Autodesk Fusion 360 part; units mm, degrees
note: some values were not read from the file. Chosen so that the rebuilt part matches the saved one: a direction. Set by a fixed rule: which sketch regions a step uses.
(part 7 of 8)
sketch "Sketch8" plane through (0, 65.3924, 0) normal (0, 1, 0) x (-1, 0, 0)
  arc A0 (-58.6914, 4.8735) -> (-58.96, 3.871) centre (-53.7044, 3) ccw
  arc A1 (-59.0732, 3.7884) -> (-58.96, 3.871) centre (-59.0587, 3.8873) ccw
  line L0 (-59.0732, 3.7884) -> (-59.8406, 3.9011)
  spline S0 degree 5 poles (-59.8406, 3.9011) (-59.8449, 3.9017) (-59.8536, 3.9029) (-59.8668, 3.9042) (-59.8844, 3.9051) (-59.9064, 3.9052) (-59.9286, 3.9045) (-59.9508, 3.9033) (-59.973, 3.9019) (-59.9953, 3.9002) (-60.0176, 3.8984) (-60.0399, 3.8963) (-60.0622, 3.8939) (-60.0846, 3.8912) (-60.107, 3.888) (-60.1294, 3.8845) (-60.1518, 3.8806) (-60.1743, 3.8765) (-60.1967, 3.8722) (-60.2192, 3.8676) (-60.2417, 3.8629) (-60.2641, 3.8579) (-60.2866, 3.8526) (-60.3091, 3.8471) (-60.3316, 3.8414) (-60.3541, 3.8354) (-60.3766, 3.8292) (-60.3991, 3.8228) (-60.4216, 3.8162) (-60.4441, 3.8093) (-60.4666, 3.8023) (-60.4891, 3.795) (-60.5116, 3.7876) (-60.5341, 3.7799) (-60.5565, 3.7721) (-60.579, 3.764) (-60.6014, 3.7558) (-60.6239, 3.7474) (-60.6463, 3.7387) (-60.6687, 3.7299) (-60.6912, 3.7209) (-60.7135, 3.7117) (-60.7359, 3.7023) (-60.7583, 3.6928) (-60.7806, 3.683) (-60.803, 3.6731) (-60.8253, 3.663) (-60.8476, 3.6527) (-60.8699, 3.6423) (-60.8921, 3.6317) (-60.9144, 3.6209) (-60.9366, 3.6099) (-60.9588, 3.5988) (-60.9809, 3.5874) (-61.0031, 3.576) (-61.0252, 3.5643) (-61.0473, 3.5525) (-61.0694, 3.5405) (-61.0914, 3.5284) (-61.1134, 3.516) (-61.1354, 3.5036) (-61.1574, 3.4909) (-61.1793, 3.4781) (-61.2012, 3.4652) (-61.2231, 3.452) (-61.2449, 3.4388) (-61.2667, 3.4253) (-61.2885, 3.4117) (-61.3102, 3.398) (-61.3319, 3.3841) (-61.3536, 3.37) (-61.3709, 3.3586) (-61.3839, 3.35) (-61.3925, 3.3443) (-61.3968, 3.3414) knots 0 0 0 0 0 0 0.01428571 0.02857143 0.04285714 0.05714286 0.07142857 0.08571429 0.1 0.11428571 0.12857143 0.14285714 0.15714286 0.17142857 0.18571429 0.2 0.21428571 0.22857143 0.24285714 0.25714286 0.27142857 0.28571429 0.3 0.31428571 0.32857143 0.34285714 0.35714286 0.37142857 0.38571429 0.4 0.41428571 0.42857143 0.44285714 0.45714286 0.47142857 0.48571429 0.5 0.51428571 0.52857143 0.54285714 0.55714286 0.57142857 0.58571429 0.6 0.61428571 0.62857143 0.64285714 0.65714286 0.67142857 0.68571429 0.7 0.71428571 0.72857143 0.74285714 0.75714286 0.77142857 0.78571429 0.8 0.81428571 0.82857143 0.84285714 0.85714286 0.87142857 0.88571429 0.9 0.91428571 0.92857143 0.94285714 0.95714286 0.97142857 0.98571429 1 1 1 1 1 1
  arc A2 (-61.3968, 3.3414) -> (-61.3968, 2.6586) centre (-53.7044, 3) ccw
  spline S1 degree 5 poles (-61.3968, 2.6586) (-61.3925, 2.6557) (-61.3839, 2.65) (-61.3709, 2.6414) (-61.3536, 2.63) (-61.3319, 2.6159) (-61.3102, 2.602) (-61.2885, 2.5883) (-61.2667, 2.5747) (-61.2449, 2.5612) (-61.2231, 2.548) (-61.2012, 2.5348) (-61.1793, 2.5219) (-61.1574, 2.5091) (-61.1354, 2.4964) (-61.1134, 2.484) (-61.0914, 2.4716) (-61.0694, 2.4595) (-61.0473, 2.4475) (-61.0252, 2.4357) (-61.0031, 2.424) (-60.9809, 2.4126) (-60.9588, 2.4012) (-60.9366, 2.3901) (-60.9144, 2.3791) (-60.8921, 2.3683) (-60.8699, 2.3577) (-60.8476, 2.3473) (-60.8253, 2.337) (-60.803, 2.3269) (-60.7806, 2.317) (-60.7583, 2.3072) (-60.7359, 2.2977) (-60.7135, 2.2883) (-60.6912, 2.2791) (-60.6687, 2.2701) (-60.6463, 2.2613) (-60.6239, 2.2526) (-60.6014, 2.2442) (-60.579, 2.236) (-60.5565, 2.2279) (-60.5341, 2.2201) (-60.5116, 2.2124) (-60.4891, 2.205) (-60.4666, 2.1977) (-60.4441, 2.1907) (-60.4216, 2.1838) (-60.3991, 2.1772) (-60.3766, 2.1708) (-60.3541, 2.1646) (-60.3316, 2.1586) (-60.3091, 2.1529) (-60.2866, 2.1474) (-60.2641, 2.1421) (-60.2417, 2.1371) (-60.2192, 2.1324) (-60.1967, 2.1278) (-60.1743, 2.1235) (-60.1518, 2.1194) (-60.1294, 2.1155) (-60.107, 2.112) (-60.0846, 2.1088) (-60.0622, 2.1061) (-60.0399, 2.1037) (-60.0176, 2.1016) (-59.9953, 2.0998) (-59.973, 2.0981) (-59.9508, 2.0967) (-59.9286, 2.0955) (-59.9064, 2.0948) (-59.8844, 2.0949) (-59.8668, 2.0958) (-59.8536, 2.0971) (-59.8449, 2.0983) (-59.8406, 2.0989) knots -1 -1 -1 -1 -1 -1 -0.98571429 -0.97142857 -0.95714286 -0.94285714 -0.92857143 -0.91428571 -0.9 -0.88571429 -0.87142857 -0.85714286 -0.84285714 -0.82857143 -0.81428571 -0.8 -0.78571429 -0.77142857 -0.75714286 -0.74285714 -0.72857143 -0.71428571 -0.7 -0.68571429 -0.67142857 -0.65714286 -0.64285714 -0.62857143 -0.61428571 -0.6 -0.58571429 -0.57142857 -0.55714286 -0.54285714 -0.52857143 -0.51428571 -0.5 -0.48571429 -0.47142857 -0.45714286 -0.44285714 -0.42857143 -0.41428571 -0.4 -0.38571429 -0.37142857 -0.35714286 -0.34285714 -0.32857143 -0.31428571 -0.3 -0.28571429 -0.27142857 -0.25714286 -0.24285714 -0.22857143 -0.21428571 -0.2 -0.18571429 -0.17142857 -0.15714286 -0.14285714 -0.12857143 -0.11428571 -0.1 -0.08571429 -0.07142857 -0.05714286 -0.04285714 -0.02857143 -0.01428571 0 0 0 0 0 0
  line L1 (-59.8406, 2.0989) -> (-59.0732, 2.2116)
  arc A3 (-58.96, 2.129) -> (-59.0732, 2.2116) centre (-59.0587, 2.1127) ccw
  arc A4 (-58.96, 2.129) -> (-58.6914, 1.1265) centre (-53.7044, 3) ccw
  arc A5 (-58.7481, 0.9984) -> (-58.6914, 1.1265) centre (-58.785, 1.0913) ccw
  line L2 (-58.7481, 0.9984) -> (-59.469, 0.7123)
  spline S2 degree 5 poles (-59.469, 0.7123) (-59.4731, 0.7106) (-59.4812, 0.7073) (-59.4933, 0.7018) (-59.5089, 0.6938) (-59.5281, 0.6829) (-59.5469, 0.6712) (-59.5656, 0.6591) (-59.5841, 0.6467) (-59.6026, 0.6342) (-59.621, 0.6215) (-59.6393, 0.6085) (-59.6574, 0.5953) (-59.6754, 0.5817) (-59.6932, 0.5677) (-59.7108, 0.5535) (-59.7283, 0.5389) (-59.7457, 0.5241) (-59.763, 0.5092) (-59.7802, 0.494) (-59.7973, 0.4786) (-59.8142, 0.463) (-59.8311, 0.4473) (-59.8478, 0.4313) (-59.8644, 0.415) (-59.8809, 0.3986) (-59.8973, 0.382) (-59.9136, 0.3652) (-59.9298, 0.3482) (-59.9458, 0.331) (-59.9618, 0.3137) (-59.9776, 0.2962) (-59.9934, 0.2785) (-60.009, 0.2606) (-60.0246, 0.2426) (-60.04, 0.2244) (-60.0553, 0.206) (-60.0705, 0.1875) (-60.0856, 0.1688) (-60.1006, 0.1499) (-60.1156, 0.1309) (-60.1304, 0.1118) (-60.145, 0.0925) (-60.1596, 0.073) (-60.1741, 0.0534) (-60.1885, 0.0336) (-60.2028, 0.0137) (-60.217, -0.0063) (-60.231, -0.0265) (-60.245, -0.0468) (-60.2588, -0.0673) (-60.2726, -0.0879) (-60.2862, -0.1087) (-60.2998, -0.1295) (-60.3132, -0.1506) (-60.3266, -0.1717) (-60.3398, -0.193) (-60.3529, -0.2144) (-60.3659, -0.2359) (-60.3788, -0.2576) (-60.3916, -0.2794) (-60.4043, -0.3013) (-60.4169, -0.3234) (-60.4294, -0.3456) (-60.4418, -0.3679) (-60.4541, -0.3903) (-60.4662, -0.4128) (-60.4783, -0.4355) (-60.4902, -0.4583) (-60.5021, -0.4812) (-60.5138, -0.5042) (-60.5231, -0.5227) (-60.53, -0.5366) (-60.5346, -0.5459) (-60.5369, -0.5506) knots 0 0 0 0 0 0 0.01428571 0.02857143 0.04285714 0.05714286 0.07142857 0.08571429 0.1 0.11428571 0.12857143 0.14285714 0.15714286 0.17142857 0.18571429 0.2 0.21428571 0.22857143 0.24285714 0.25714286 0.27142857 0.28571429 0.3 0.31428571 0.32857143 0.34285714 0.35714286 0.37142857 0.38571429 0.4 0.41428571 0.42857143 0.44285714 0.45714286 0.47142857 0.48571429 0.5 0.51428571 0.52857143 0.54285714 0.55714286 0.57142857 0.58571429 0.6 0.61428571 0.62857143 0.64285714 0.65714286 0.67142857 0.68571429 0.7 0.71428571 0.72857143 0.74285714 0.75714286 0.77142857 0.78571429 0.8 0.81428571 0.82857143 0.84285714 0.85714286 0.87142857 0.88571429 0.9 0.91428571 0.92857143 0.94285714 0.95714286 0.97142857 0.98571429 1 1 1 1 1 1
  arc A6 (-60.5369, -0.5506) -> (-60.1955, -1.1419) centre (-53.7044, 3) ccw
  spline S3 degree 5 poles (-60.1955, -1.1419) (-60.1904, -1.1422) (-60.18, -1.1429) (-60.1645, -1.1438) (-60.1438, -1.145) (-60.118, -1.1464) (-60.0922, -1.1476) (-60.0665, -1.1486) (-60.0409, -1.1495) (-60.0153, -1.1502) (-59.9897, -1.1508) (-59.9642, -1.1513) (-59.9388, -1.1515) (-59.9134, -1.1516) (-59.8881, -1.1516) (-59.8628, -1.1514) (-59.8376, -1.1511) (-59.8124, -1.1506) (-59.7873, -1.1499) (-59.7622, -1.1491) (-59.7373, -1.1481) (-59.7123, -1.147) (-59.6875, -1.1457) (-59.6627, -1.1443) (-59.638, -1.1427) (-59.6133, -1.1409) (-59.5887, -1.139) (-59.5642, -1.1369) (-59.5398, -1.1346) (-59.5154, -1.1322) (-59.4911, -1.1297) (-59.4669, -1.1269) (-59.4427, -1.124) (-59.4186, -1.1209) (-59.3947, -1.1177) (-59.3707, -1.1143) (-59.3469, -1.1107) (-59.3232, -1.107) (-59.2995, -1.1031) (-59.2759, -1.099) (-59.2525, -1.0947) (-59.2291, -1.0903) (-59.2058, -1.0857) (-59.1826, -1.0809) (-59.1595, -1.0759) (-59.1365, -1.0708) (-59.1136, -1.0654) (-59.0908, -1.0599) (-59.0681, -1.0542) (-59.0455, -1.0483) (-59.023, -1.0423) (-59.0007, -1.036) (-58.9785, -1.0295) (-58.9564, -1.0228) (-58.9344, -1.0159) (-58.9126, -1.0088) (-58.8908, -1.0015) (-58.8692, -0.994) (-58.8477, -0.9864) (-58.8264, -0.9785) (-58.8052, -0.9703) (-58.7842, -0.9619) (-58.7635, -0.9531) (-58.7429, -0.944) (-58.7226, -0.9346) (-58.7023, -0.9251) (-58.6823, -0.9154) (-58.6623, -0.9055) (-58.6425, -0.8954) (-58.6229, -0.8849) (-58.6039, -0.8738) (-58.5891, -0.8642) (-58.5784, -0.8565) (-58.5714, -0.8512) (-58.5679, -0.8484) knots -1 -1 -1 -1 -1 -1 -0.98571429 -0.97142857 -0.95714286 -0.94285714 -0.92857143 -0.91428571 -0.9 -0.88571429 -0.87142857 -0.85714286 -0.84285714 -0.82857143 -0.81428571 -0.8 -0.78571429 -0.77142857 -0.75714286 -0.74285714 -0.72857143 -0.71428571 -0.7 -0.68571429 -0.67142857 -0.65714286 -0.64285714 -0.62857143 -0.61428571 -0.6 -0.58571429 -0.57142857 -0.55714286 -0.54285714 -0.52857143 -0.51428571 -0.5 -0.48571429 -0.47142857 -0.45714286 -0.44285714 -0.42857143 -0.41428571 -0.4 -0.38571429 -0.37142857 -0.35714286 -0.34285714 -0.32857143 -0.31428571 -0.3 -0.28571429 -0.27142857 -0.25714286 -0.24285714 -0.22857143 -0.21428571 -0.2 -0.18571429 -0.17142857 -0.15714286 -0.14285714 -0.12857143 -0.11428571 -0.1 -0.08571429 -0.07142857 -0.05714286 -0.04285714 -0.02857143 -0.01428571 0 0 0 0 0 0
  line L3 (-58.5679, -0.8484) -> (-57.9597, -0.3672)
  arc A7 (-57.8204, -0.3821) -> (-57.9597, -0.3672) centre (-57.8977, -0.4456) ccw
  arc A8 (-57.8204, -0.3821) -> (-57.0865, -1.116) centre (-53.7044, 3) ccw
  arc A9 (-57.0716, -1.2553) -> (-57.0865, -1.116) centre (-57.15, -1.1933) ccw
  line L4 (-57.0716, -1.2553) -> (-57.5528, -1.8635)
  spline S4 degree 5 poles (-57.5528, -1.8635) (-57.5556, -1.867) (-57.5609, -1.874) (-57.5686, -1.8847) (-57.5782, -1.8995) (-57.5893, -1.9185) (-57.5998, -1.9381) (-57.6099, -1.9579) (-57.6197, -1.9779) (-57.6295, -1.998) (-57.639, -2.0182) (-57.6484, -2.0385) (-57.6575, -2.0591) (-57.6663, -2.0798) (-57.6747, -2.1008) (-57.6829, -2.122) (-57.6908, -2.1433) (-57.6984, -2.1648) (-57.7059, -2.1864) (-57.7132, -2.2082) (-57.7203, -2.23) (-57.7272, -2.252) (-57.7339, -2.2741) (-57.7404, -2.2963) (-57.7467, -2.3187) (-57.7527, -2.3411) (-57.7586, -2.3637) (-57.7643, -2.3864) (-57.7698, -2.4092) (-57.7751, -2.4321) (-57.7803, -2.4551) (-57.7853, -2.4782) (-57.7901, -2.5014) (-57.7947, -2.5247) (-57.7991, -2.5481) (-57.8034, -2.5716) (-57.8075, -2.5951) (-57.8114, -2.6188) (-57.8151, -2.6425) (-57.8187, -2.6664) (-57.8221, -2.6903) (-57.8253, -2.7143) (-57.8284, -2.7383) (-57.8313, -2.7625) (-57.834, -2.7867) (-57.8366, -2.811) (-57.839, -2.8354) (-57.8413, -2.8598) (-57.8434, -2.8843) (-57.8453, -2.9089) (-57.8471, -2.9336) (-57.8487, -2.9583) (-57.8501, -2.9831) (-57.8514, -3.008) (-57.8525, -3.0329) (-57.8535, -3.0579) (-57.8543, -3.0829) (-57.855, -3.108) (-57.8555, -3.1332) (-57.8558, -3.1584) (-57.856, -3.1837) (-57.856, -3.209) (-57.8559, -3.2344) (-57.8556, -3.2599) (-57.8552, -3.2854) (-57.8546, -3.3109) (-57.8539, -3.3365) (-57.853, -3.3622) (-57.852, -3.3879) (-57.8508, -3.4136) (-57.8494, -3.4394) (-57.8482, -3.4601) (-57.8473, -3.4756) (-57.8466, -3.486) (-57.8462, -3.4911) knots 0 0 0 0 0 0 0.01428571 0.02857143 0.04285714 0.05714286 0.07142857 0.08571429 0.1 0.11428571 0.12857143 0.14285714 0.15714286 0.17142857 0.18571429 0.2 0.21428571 0.22857143 0.24285714 0.25714286 0.27142857 0.28571429 0.3 0.31428571 0.32857143 0.34285714 0.35714286 0.37142857 0.38571429 0.4 0.41428571 0.42857143 0.44285714 0.45714286 0.47142857 0.48571429 0.5 0.51428571 0.52857143 0.54285714 0.55714286 0.57142857 0.58571429 0.6 0.61428571 0.62857143 0.64285714 0.65714286 0.67142857 0.68571429 0.7 0.71428571 0.72857143 0.74285714 0.75714286 0.77142857 0.78571429 0.8 0.81428571 0.82857143 0.84285714 0.85714286 0.87142857 0.88571429 0.9 0.91428571 0.92857143 0.94285714 0.95714286 0.97142857 0.98571429 1 1 1 1 1 1
  arc A10 (-57.8462, -3.4911) -> (-57.255, -3.8325) centre (-53.7044, 3) ccw
  spline S5 degree 5 poles (-57.255, -3.8325) (-57.2503, -3.8302) (-57.241, -3.8256) (-57.2271, -3.8187) (-57.2086, -3.8094) (-57.1855, -3.7977) (-57.1626, -3.7858) (-57.1399, -3.7739) (-57.1172, -3.7618) (-57.0947, -3.7497) (-57.0723, -3.7374) (-57.05, -3.725) (-57.0278, -3.7125) (-57.0057, -3.6999) (-56.9838, -3.6872) (-56.962, -3.6744) (-56.9403, -3.6615) (-56.9188, -3.6485) (-56.8974, -3.6354) (-56.8761, -3.6222) (-56.8549, -3.6088) (-56.8339, -3.5954) (-56.813, -3.5819) (-56.7923, -3.5682) (-56.7717, -3.5545) (-56.7512, -3.5406) (-56.7309, -3.5266) (-56.7107, -3.5126) (-56.6906, -3.4984) (-56.6707, -3.4841) (-56.651, -3.4697) (-56.6314, -3.4552) (-56.6119, -3.4407) (-56.5926, -3.426) (-56.5735, -3.4112) (-56.5544, -3.3963) (-56.5356, -3.3813) (-56.5169, -3.3661) (-56.4984, -3.3509) (-56.48, -3.3356) (-56.4618, -3.3202) (-56.4438, -3.3046) (-56.4259, -3.289) (-56.4082, -3.2732) (-56.3907, -3.2574) (-56.3734, -3.2414) (-56.3562, -3.2254) (-56.3392, -3.2092) (-56.3224, -3.1929) (-56.3058, -3.1765) (-56.2893, -3.16) (-56.2731, -3.1434) (-56.2571, -3.1267) (-56.2413, -3.1098) (-56.2258, -3.0929) (-56.2104, -3.0758) (-56.1952, -3.0586) (-56.1802, -3.0413) (-56.1655, -3.024) (-56.1509, -3.0065) (-56.1367, -2.9888) (-56.1227, -2.971) (-56.1091, -2.953) (-56.0959, -2.9349) (-56.0829, -2.9166) (-56.0702, -2.8982) (-56.0577, -2.8797) (-56.0453, -2.8612) (-56.0332, -2.8426) (-56.0215, -2.8237) (-56.0105, -2.8046) (-56.0026, -2.7889) (-55.9971, -2.7768) (-55.9937, -2.7687) (-55.9921, -2.7646) knots -1 -1 -1 -1 -1 -1 -0.98571429 -0.97142857 -0.95714286 -0.94285714 -0.92857143 -0.91428571 -0.9 -0.88571429 -0.87142857 -0.85714286 -0.84285714 -0.82857143 -0.81428571 -0.8 -0.78571429 -0.77142857 -0.75714286 -0.74285714 -0.72857143 -0.71428571 -0.7 -0.68571429 -0.67142857 -0.65714286 -0.64285714 -0.62857143 -0.61428571 -0.6 -0.58571429 -0.57142857 -0.55714286 -0.54285714 -0.52857143 -0.51428571 -0.5 -0.48571429 -0.47142857 -0.45714286 -0.44285714 -0.42857143 -0.41428571 -0.4 -0.38571429 -0.37142857 -0.35714286 -0.34285714 -0.32857143 -0.31428571 -0.3 -0.28571429 -0.27142857 -0.25714286 -0.24285714 -0.22857143 -0.21428571 -0.2 -0.18571429 -0.17142857 -0.15714286 -0.14285714 -0.12857143 -0.11428571 -0.1 -0.08571429 -0.07142857 -0.05714286 -0.04285714 -0.02857143 -0.01428571 0 0 0 0 0 0
  line L5 (-55.9921, -2.7646) -> (-55.706, -2.0437)
  arc A11 (-55.5779, -1.987) -> (-55.706, -2.0437) centre (-55.6131, -2.0806) ccw
  arc A12 (-55.5779, -1.987) -> (-54.5754, -2.2556) centre (-53.7044, 3) ccw
  arc A13 (-54.4928, -2.3688) -> (-54.5754, -2.2556) centre (-54.5917, -2.3543) ccw
  line L6 (-54.4928, -2.3688) -> (-54.6055, -3.1362)
  spline S6 degree 5 poles (-54.6055, -3.1362) (-54.6061, -3.1405) (-54.6072, -3.1493) (-54.6085, -3.1624) (-54.6095, -3.18) (-54.6096, -3.202) (-54.6089, -3.2242) (-54.6077, -3.2464) (-54.6063, -3.2686) (-54.6046, -3.2909) (-54.6028, -3.3132) (-54.6007, -3.3355) (-54.5983, -3.3578) (-54.5956, -3.3802) (-54.5924, -3.4026) (-54.5889, -3.425) (-54.585, -3.4474) (-54.5809, -3.4699) (-54.5766, -3.4923) (-54.572, -3.5148) (-54.5672, -3.5373) (-54.5622, -3.5598) (-54.557, -3.5822) (-54.5515, -3.6047) (-54.5458, -3.6272) (-54.5398, -3.6497) (-54.5336, -3.6722) (-54.5272, -3.6947) (-54.5205, -3.7172) (-54.5137, -3.7397) (-54.5067, -3.7622) (-54.4994, -3.7847) (-54.492, -3.8072) (-54.4843, -3.8297) (-54.4765, -3.8521) (-54.4684, -3.8746) (-54.4602, -3.8971) (-54.4517, -3.9195) (-54.4431, -3.9419) (-54.4343, -3.9644) (-54.4253, -3.9868) (-54.4161, -4.0092) (-54.4067, -4.0315) (-54.3972, -4.0539) (-54.3874, -4.0763) (-54.3775, -4.0986) (-54.3674, -4.1209) (-54.3571, -4.1432) (-54.3467, -4.1655) (-54.3361, -4.1877) (-54.3253, -4.21) (-54.3143, -4.2322) (-54.3031, -4.2544) (-54.2918, -4.2765) (-54.2803, -4.2987) (-54.2687, -4.3208) (-54.2569, -4.3429) (-54.2449, -4.365) (-54.2327, -4.387) (-54.2204, -4.409) (-54.208, -4.431) (-54.1953, -4.453) (-54.1825, -4.4749) (-54.1696, -4.4968) (-54.1564, -4.5187) (-54.1432, -4.5405) (-54.1297, -4.5623) (-54.1161, -4.5841) (-54.1024, -4.6058) (-54.0885, -4.6275) (-54.0744, -4.6492) (-54.063, -4.6665) (-54.0544, -4.6795) (-54.0487, -4.6881) (-54.0458, -4.6924) knots 0 0 0 0 0 0 0.01428571 0.02857143 0.04285714 0.05714286 0.07142857 0.08571429 0.1 0.11428571 0.12857143 0.14285714 0.15714286 0.17142857 0.18571429 0.2 0.21428571 0.22857143 0.24285714 0.25714286 0.27142857 0.28571429 0.3 0.31428571 0.32857143 0.34285714 0.35714286 0.37142857 0.38571429 0.4 0.41428571 0.42857143 0.44285714 0.45714286 0.47142857 0.48571429 0.5 0.51428571 0.52857143 0.54285714 0.55714286 0.57142857 0.58571429 0.6 0.61428571 0.62857143 0.64285714 0.65714286 0.67142857 0.68571429 0.7 0.71428571 0.72857143 0.74285714 0.75714286 0.77142857 0.78571429 0.8 0.81428571 0.82857143 0.84285714 0.85714286 0.87142857 0.88571429 0.9 0.91428571 0.92857143 0.94285714 0.95714286 0.97142857 0.98571429 1 1 1 1 1 1
  arc A14 (-54.0458, -4.6924) -> (-53.363, -4.6924) centre (-53.7044, 3) ccw
  spline S7 degree 5 poles (-53.363, -4.6924) (-53.3601, -4.6881) (-53.3544, -4.6795) (-53.3458, -4.6665) (-53.3344, -4.6492) (-53.3203, -4.6275) (-53.3064, -4.6058) (-53.2927, -4.5841) (-53.2791, -4.5623) (-53.2656, -4.5405) (-53.2523, -4.5187) (-53.2392, -4.4968) (-53.2263, -4.4749) (-53.2135, -4.453) (-53.2008, -4.431) (-53.1883, -4.409) (-53.176, -4.387) (-53.1639, -4.365) (-53.1519, -4.3429) (-53.1401, -4.3208) (-53.1284, -4.2987) (-53.117, -4.2765) (-53.1056, -4.2544) (-53.0945, -4.2322) (-53.0835, -4.21) (-53.0727, -4.1877) (-53.0621, -4.1655) (-53.0516, -4.1432) (-53.0414, -4.1209) (-53.0313, -4.0986) (-53.0213, -4.0763) (-53.0116, -4.0539) (-53.0021, -4.0315) (-52.9927, -4.0092) (-52.9835, -3.9868) (-52.9745, -3.9644) (-52.9657, -3.9419) (-52.957, -3.9195) (-52.9486, -3.8971) (-52.9403, -3.8746) (-52.9323, -3.8521) (-52.9244, -3.8297) (-52.9168, -3.8072) (-52.9093, -3.7847) (-52.9021, -3.7622) (-52.8951, -3.7397) (-52.8882, -3.7172) (-52.8816, -3.6947) (-52.8752, -3.6722) (-52.869, -3.6497) (-52.863, -3.6272) (-52.8573, -3.6047) (-52.8518, -3.5822) (-52.8465, -3.5598) (-52.8415, -3.5373) (-52.8368, -3.5148) (-52.8322, -3.4923) (-52.8279, -3.4699) (-52.8238, -3.4474) (-52.8199, -3.425) (-52.8164, -3.4026) (-52.8132, -3.3802) (-52.8104, -3.3578) (-52.808, -3.3355) (-52.806, -3.3132) (-52.8042, -3.2909) (-52.8025, -3.2686) (-52.8011, -3.2464) (-52.7999, -3.2242) (-52.7992, -3.202) (-52.7993, -3.18) (-52.8002, -3.1624) (-52.8015, -3.1493) (-52.8027, -3.1405) (-52.8033, -3.1362) knots -1 -1 -1 -1 -1 -1 -0.98571429 -0.97142857 -0.95714286 -0.94285714 -0.92857143 -0.91428571 -0.9 -0.88571429 -0.87142857 -0.85714286 -0.84285714 -0.82857143 -0.81428571 -0.8 -0.78571429 -0.77142857 -0.75714286 -0.74285714 -0.72857143 -0.71428571 -0.7 -0.68571429 -0.67142857 -0.65714286 -0.64285714 -0.62857143 -0.61428571 -0.6 -0.58571429 -0.57142857 -0.55714286 -0.54285714 -0.52857143 -0.51428571 -0.5 -0.48571429 -0.47142857 -0.45714286 -0.44285714 -0.42857143 -0.41428571 -0.4 -0.38571429 -0.37142857 -0.35714286 -0.34285714 -0.32857143 -0.31428571 -0.3 -0.28571429 -0.27142857 -0.25714286 -0.24285714 -0.22857143 -0.21428571 -0.2 -0.18571429 -0.17142857 -0.15714286 -0.14285714 -0.12857143 -0.11428571 -0.1 -0.08571429 -0.07142857 -0.05714286 -0.04285714 -0.02857143 -0.01428571 0 0 0 0 0 0
  line L7 (-52.8033, -3.1362) -> (-52.916, -2.3688)
  arc A15 (-52.8334, -2.2556) -> (-52.916, -2.3688) centre (-52.8171, -2.3543) ccw
  arc A16 (-52.8334, -2.2556) -> (-51.8309, -1.987) centre (-53.7044, 3) ccw
  arc A17 (-51.7028, -2.0437) -> (-51.8309, -1.987) centre (-51.7957, -2.0806) ccw
  line L8 (-51.7028, -2.0437) -> (-51.4167, -2.7646)
  spline S8 degree 5 poles (-51.4167, -2.7646) (-51.415, -2.7687) (-51.4117, -2.7768) (-51.4062, -2.7889) (-51.3982, -2.8046) (-51.3873, -2.8237) (-51.3756, -2.8426) (-51.3635, -2.8612) (-51.3511, -2.8797) (-51.3386, -2.8982) (-51.3258, -2.9166) (-51.3129, -2.9349) (-51.2997, -2.953) (-51.2861, -2.971) (-51.2721, -2.9888) (-51.2579, -3.0065) (-51.2433, -3.024) (-51.2285, -3.0413) (-51.2135, -3.0586) (-51.1984, -3.0758) (-51.183, -3.0929) (-51.1674, -3.1098) (-51.1517, -3.1267) (-51.1356, -3.1434) (-51.1194, -3.16) (-51.103, -3.1765) (-51.0864, -3.1929) (-51.0696, -3.2092) (-51.0526, -3.2254) (-51.0354, -3.2414) (-51.0181, -3.2574) (-51.0006, -3.2732) (-50.9829, -3.289) (-50.965, -3.3046) (-50.947, -3.3202) (-50.9288, -3.3356) (-50.9104, -3.3509) (-50.8919, -3.3661) (-50.8732, -3.3813) (-50.8543, -3.3963) (-50.8353, -3.4112) (-50.8162, -3.426) (-50.7969, -3.4407) (-50.7774, -3.4552) (-50.7578, -3.4697) (-50.738, -3.4841) (-50.7181, -3.4984) (-50.6981, -3.5126) (-50.6779, -3.5266) (-50.6576, -3.5406) (-50.6371, -3.5545) (-50.6165, -3.5682) (-50.5957, -3.5819) (-50.5749, -3.5954) (-50.5538, -3.6088) (-50.5327, -3.6222) (-50.5114, -3.6354) (-50.49, -3.6485) (-50.4684, -3.6615) (-50.4468, -3.6744) (-50.425, -3.6872) (-50.403, -3.6999) (-50.381, -3.7125) (-50.3588, -3.725) (-50.3365, -3.7374) (-50.3141, -3.7497) (-50.2916, -3.7618) (-50.2689, -3.7739) (-50.2461, -3.7858) (-50.2232, -3.7977) (-50.2002, -3.8094) (-50.1817, -3.8187) (-50.1678, -3.8256) (-50.1585, -3.8302) (-50.1538, -3.8325) knots 0 0 0 0 0 0 0.01428571 0.02857143 0.04285714 0.05714286 0.07142857 0.08571429 0.1 0.11428571 0.12857143 0.14285714 0.15714286 0.17142857 0.18571429 0.2 0.21428571 0.22857143 0.24285714 0.25714286 0.27142857 0.28571429 0.3 0.31428571 0.32857143 0.34285714 0.35714286 0.37142857 0.38571429 0.4 0.41428571 0.42857143 0.44285714 0.45714286 0.47142857 0.48571429 0.5 0.51428571 0.52857143 0.54285714 0.55714286 0.57142857 0.58571429 0.6 0.61428571 0.62857143 0.64285714 0.65714286 0.67142857 0.68571429 0.7 0.71428571 0.72857143 0.74285714 0.75714286 0.77142857 0.78571429 0.8 0.81428571 0.82857143 0.84285714 0.85714286 0.87142857 0.88571429 0.9 0.91428571 0.92857143 0.94285714 0.95714286 0.97142857 0.98571429 1 1 1 1 1 1
  arc A18 (-50.1538, -3.8325) -> (-49.5625, -3.4911) centre (-53.7044, 3) ccw
  spline S9 degree 5 poles (-49.5625, -3.4911) (-49.5622, -3.486) (-49.5615, -3.4756) (-49.5605, -3.4601) (-49.5593, -3.4394) (-49.558, -3.4136) (-49.5568, -3.3879) (-49.5558, -3.3622) (-49.5549, -3.3365) (-49.5541, -3.3109) (-49.5536, -3.2854) (-49.5531, -3.2599) (-49.5529, -3.2344) (-49.5527, -3.209) (-49.5528, -3.1837) (-49.553, -3.1584) (-49.5533, -3.1332) (-49.5538, -3.108) (-49.5545, -3.0829) (-49.5553, -3.0579) (-49.5562, -3.0329) (-49.5574, -3.008) (-49.5587, -2.9831) (-49.5601, -2.9583) (-49.5617, -2.9336) (-49.5635, -2.9089) (-49.5654, -2.8843) (-49.5675, -2.8598) (-49.5697, -2.8354) (-49.5722, -2.811) (-49.5747, -2.7867) (-49.5775, -2.7625) (-49.5804, -2.7383) (-49.5834, -2.7143) (-49.5867, -2.6903) (-49.5901, -2.6664) (-49.5937, -2.6425) (-49.5974, -2.6188) (-49.6013, -2.5951) (-49.6054, -2.5716) (-49.6097, -2.5481) (-49.6141, -2.5247) (-49.6187, -2.5014) (-49.6235, -2.4782) (-49.6285, -2.4551) (-49.6336, -2.4321) (-49.639, -2.4092) (-49.6445, -2.3864) (-49.6502, -2.3637) (-49.656, -2.3411) (-49.6621, -2.3187) (-49.6684, -2.2963) (-49.6749, -2.2741) (-49.6816, -2.252) (-49.6885, -2.23) (-49.6956, -2.2082) (-49.7029, -2.1864) (-49.7104, -2.1648) (-49.718, -2.1433) (-49.7259, -2.122) (-49.7341, -2.1008) (-49.7425, -2.0798) (-49.7513, -2.0591) (-49.7604, -2.0385) (-49.7697, -2.0182) (-49.7793, -1.998) (-49.789, -1.9779) (-49.7989, -1.9579) (-49.809, -1.9381) (-49.8195, -1.9185) (-49.8306, -1.8995) (-49.8402, -1.8847) (-49.8479, -1.874) (-49.8532, -1.867) (-49.856, -1.8635) knots -1 -1 -1 -1 -1 -1 -0.98571429 -0.97142857 -0.95714286 -0.94285714 -0.92857143 -0.91428571 -0.9 -0.88571429 -0.87142857 -0.85714286 -0.84285714 -0.82857143 -0.81428571 -0.8 -0.78571429 -0.77142857 -0.75714286 -0.74285714 -0.72857143 -0.71428571 -0.7 -0.68571429 -0.67142857 -0.65714286 -0.64285714 -0.62857143 -0.61428571 -0.6 -0.58571429 -0.57142857 -0.55714286 -0.54285714 -0.52857143 -0.51428571 -0.5 -0.48571429 -0.47142857 -0.45714286 -0.44285714 -0.42857143 -0.41428571 -0.4 -0.38571429 -0.37142857 -0.35714286 -0.34285714 -0.32857143 -0.31428571 -0.3 -0.28571429 -0.27142857 -0.25714286 -0.24285714 -0.22857143 -0.21428571 -0.2 -0.18571429 -0.17142857 -0.15714286 -0.14285714 -0.12857143 -0.11428571 -0.1 -0.08571429 -0.07142857 -0.05714286 -0.04285714 -0.02857143 -0.01428571 0 0 0 0 0 0
  line L9 (-49.856, -1.8635) -> (-50.3372, -1.2553)
  arc A19 (-50.3223, -1.116) -> (-50.3372, -1.2553) centre (-50.2588, -1.1933) ccw
  arc A20 (-50.3223, -1.116) -> (-49.5884, -0.3821) centre (-53.7044, 3) ccw
  arc A21 (-49.4491, -0.3672) -> (-49.5884, -0.3821) centre (-49.5111, -0.4456) ccw
  line L10 (-49.4491, -0.3672) -> (-48.8409, -0.8484)
  spline S10 degree 5 poles (-48.8409, -0.8484) (-48.8374, -0.8512) (-48.8304, -0.8565) (-48.8197, -0.8642) (-48.8049, -0.8738) (-48.7859, -0.8849) (-48.7663, -0.8954) (-48.7465, -0.9055) (-48.7265, -0.9154) (-48.7064, -0.9251) (-48.6862, -0.9346) (-48.6659, -0.944) (-48.6453, -0.9531) (-48.6246, -0.9619) (-48.6036, -0.9703) (-48.5824, -0.9785) (-48.5611, -0.9864) (-48.5396, -0.994) (-48.5179, -1.0015) (-48.4962, -1.0088) (-48.4744, -1.0159) (-48.4524, -1.0228) (-48.4303, -1.0295) (-48.4081, -1.036) (-48.3857, -1.0423) (-48.3633, -1.0483) (-48.3407, -1.0542) (-48.318, -1.0599) (-48.2952, -1.0654) (-48.2723, -1.0708) (-48.2493, -1.0759) (-48.2262, -1.0809) (-48.203, -1.0857) (-48.1797, -1.0903) (-48.1563, -1.0947) (-48.1328, -1.099) (-48.1093, -1.1031) (-48.0856, -1.107) (-48.0619, -1.1107) (-48.038, -1.1143) (-48.0141, -1.1177) (-47.9901, -1.1209) (-47.9661, -1.124) (-47.9419, -1.1269) (-47.9177, -1.1297) (-47.8934, -1.1322) (-47.869, -1.1346) (-47.8446, -1.1369) (-47.8201, -1.139) (-47.7955, -1.1409) (-47.7708, -1.1427) (-47.7461, -1.1443) (-47.7213, -1.1457) (-47.6964, -1.147) (-47.6715, -1.1481) (-47.6465, -1.1491) (-47.6215, -1.1499) (-47.5964, -1.1506) (-47.5712, -1.1511) (-47.546, -1.1514) (-47.5207, -1.1516) (-47.4954, -1.1516) (-47.47, -1.1515) (-47.4445, -1.1513) (-47.419, -1.1508) (-47.3935, -1.1502) (-47.3679, -1.1495) (-47.3422, -1.1486) (-47.3165, -1.1476) (-47.2908, -1.1464) (-47.265, -1.145) (-47.2443, -1.1438) (-47.2288, -1.1429) (-47.2184, -1.1422) (-47.2132, -1.1419) knots 0 0 0 0 0 0 0.01428571 0.02857143 0.04285714 0.05714286 0.07142857 0.08571429 0.1 0.11428571 0.12857143 0.14285714 0.15714286 0.17142857 0.18571429 0.2 0.21428571 0.22857143 0.24285714 0.25714286 0.27142857 0.28571429 0.3 0.31428571 0.32857143 0.34285714 0.35714286 0.37142857 0.38571429 0.4 0.41428571 0.42857143 0.44285714 0.45714286 0.47142857 0.48571429 0.5 0.51428571 0.52857143 0.54285714 0.55714286 0.57142857 0.58571429 0.6 0.61428571 0.62857143 0.64285714 0.65714286 0.67142857 0.68571429 0.7 0.71428571 0.72857143 0.74285714 0.75714286 0.77142857 0.78571429 0.8 0.81428571 0.82857143 0.84285714 0.85714286 0.87142857 0.88571429 0.9 0.91428571 0.92857143 0.94285714 0.95714286 0.97142857 0.98571429 1 1 1 1 1 1
  arc A22 (-47.2132, -1.1419) -> (-46.8719, -0.5506) centre (-53.7044, 3) ccw
  spline S11 degree 5 poles (-46.8719, -0.5506) (-46.8742, -0.5459) (-46.8787, -0.5366) (-46.8857, -0.5227) (-46.895, -0.5042) (-46.9067, -0.4812) (-46.9186, -0.4583) (-46.9305, -0.4355) (-46.9426, -0.4128) (-46.9547, -0.3903) (-46.967, -0.3679) (-46.9794, -0.3456) (-46.9919, -0.3234) (-47.0044, -0.3013) (-47.0171, -0.2794) (-47.0299, -0.2576) (-47.0429, -0.2359) (-47.0559, -0.2144) (-47.069, -0.193) (-47.0822, -0.1717) (-47.0956, -0.1506) (-47.109, -0.1295) (-47.1225, -0.1087) (-47.1362, -0.0879) (-47.1499, -0.0673) (-47.1638, -0.0468) (-47.1778, -0.0265) (-47.1918, -0.0063) (-47.206, 0.0137) (-47.2203, 0.0336) (-47.2347, 0.0534) (-47.2491, 0.073) (-47.2637, 0.0925) (-47.2784, 0.1118) (-47.2932, 0.1309) (-47.3081, 0.1499) (-47.3231, 0.1688) (-47.3382, 0.1875) (-47.3535, 0.206) (-47.3688, 0.2244) (-47.3842, 0.2426) (-47.3997, 0.2606) (-47.4154, 0.2785) (-47.4311, 0.2962) (-47.447, 0.3137) (-47.463, 0.331) (-47.479, 0.3482) (-47.4952, 0.3652) (-47.5115, 0.382) (-47.5279, 0.3986) (-47.5443, 0.415) (-47.561, 0.4313) (-47.5777, 0.4473) (-47.5945, 0.463) (-47.6115, 0.4786) (-47.6286, 0.494) (-47.6458, 0.5092) (-47.663, 0.5241) (-47.6804, 0.5389) (-47.6979, 0.5535) (-47.7156, 0.5677) (-47.7334, 0.5817) (-47.7514, 0.5953) (-47.7695, 0.6085) (-47.7878, 0.6215) (-47.8062, 0.6342) (-47.8247, 0.6467) (-47.8432, 0.6591) (-47.8618, 0.6712) (-47.8807, 0.6829) (-47.8998, 0.6938) (-47.9155, 0.7018) (-47.9275, 0.7073) (-47.9357, 0.7106) (-47.9398, 0.7123) knots -1 -1 -1 -1 -1 -1 -0.98571429 -0.97142857 -0.95714286 -0.94285714 -0.92857143 -0.91428571 -0.9 -0.88571429 -0.87142857 -0.85714286 -0.84285714 -0.82857143 -0.81428571 -0.8 -0.78571429 -0.77142857 -0.75714286 -0.74285714 -0.72857143 -0.71428571 -0.7 -0.68571429 -0.67142857 -0.65714286 -0.64285714 -0.62857143 -0.61428571 -0.6 -0.58571429 -0.57142857 -0.55714286 -0.54285714 -0.52857143 -0.51428571 -0.5 -0.48571429 -0.47142857 -0.45714286 -0.44285714 -0.42857143 -0.41428571 -0.4 -0.38571429 -0.37142857 -0.35714286 -0.34285714 -0.32857143 -0.31428571 -0.3 -0.28571429 -0.27142857 -0.25714286 -0.24285714 -0.22857143 -0.21428571 -0.2 -0.18571429 -0.17142857 -0.15714286 -0.14285714 -0.12857143 -0.11428571 -0.1 -0.08571429 -0.07142857 -0.05714286 -0.04285714 -0.02857143 -0.01428571 0 0 0 0 0 0
  line L11 (-47.9398, 0.7123) -> (-48.6607, 0.9984)
  arc A23 (-48.7174, 1.1265) -> (-48.6607, 0.9984) centre (-48.6238, 1.0913) ccw
  arc A24 (-48.7174, 1.1265) -> (-48.4488, 2.129) centre (-53.7044, 3) ccw
  arc A25 (-48.3356, 2.2116) -> (-48.4488, 2.129) centre (-48.3501, 2.1127) ccw
  line L12 (-48.3356, 2.2116) -> (-47.5682, 2.0989)
  spline S12 degree 5 poles (-47.5682, 2.0989) (-47.5639, 2.0983) (-47.5551, 2.0971) (-47.542, 2.0958) (-47.5244, 2.0949) (-47.5023, 2.0948) (-47.4802, 2.0955) (-47.458, 2.0967) (-47.4358, 2.0981) (-47.4135, 2.0998) (-47.3912, 2.1016) (-47.3689, 2.1037) (-47.3465, 2.1061) (-47.3242, 2.1088) (-47.3018, 2.112) (-47.2794, 2.1155) (-47.2569, 2.1194) (-47.2345, 2.1235) (-47.212, 2.1278) (-47.1896, 2.1324) (-47.1671, 2.1371) (-47.1446, 2.1421) (-47.1221, 2.1474) (-47.0997, 2.1529) (-47.0772, 2.1586) (-47.0547, 2.1646) (-47.0322, 2.1708) (-47.0097, 2.1772) (-46.9872, 2.1838) (-46.9647, 2.1907) (-46.9422, 2.1977) (-46.9197, 2.205) (-46.8972, 2.2124) (-46.8747, 2.2201) (-46.8523, 2.2279) (-46.8298, 2.236) (-46.8073, 2.2442) (-46.7849, 2.2526) (-46.7625, 2.2613) (-46.74, 2.2701) (-46.7176, 2.2791) (-46.6952, 2.2883) (-46.6729, 2.2977) (-46.6505, 2.3072) (-46.6281, 2.317) (-46.6058, 2.3269) (-46.5835, 2.337) (-46.5612, 2.3473) (-46.5389, 2.3577) (-46.5167, 2.3683) (-46.4944, 2.3791) (-46.4722, 2.3901) (-46.45, 2.4012) (-46.4278, 2.4126) (-46.4057, 2.424) (-46.3836, 2.4357) (-46.3615, 2.4475) (-46.3394, 2.4595) (-46.3174, 2.4716) (-46.2953, 2.484) (-46.2734, 2.4964) (-46.2514, 2.5091) (-46.2295, 2.5219) (-46.2076, 2.5348) (-46.1857, 2.548) (-46.1639, 2.5612) (-46.1421, 2.5747) (-46.1203, 2.5883) (-46.0986, 2.602) (-46.0769, 2.6159) (-46.0552, 2.63) (-46.0379, 2.6414) (-46.0249, 2.65) (-46.0163, 2.6557) (-46.012, 2.6586) knots 0 0 0 0 0 0 0.01428571 0.02857143 0.04285714 0.05714286 0.07142857 0.08571429 0.1 0.11428571 0.12857143 0.14285714 0.15714286 0.17142857 0.18571429 0.2 0.21428571 0.22857143 0.24285714 0.25714286 0.27142857 0.28571429 0.3 0.31428571 0.32857143 0.34285714 0.35714286 0.37142857 0.38571429 0.4 0.41428571 0.42857143 0.44285714 0.45714286 0.47142857 0.48571429 0.5 0.51428571 0.52857143 0.54285714 0.55714286 0.57142857 0.58571429 0.6 0.61428571 0.62857143 0.64285714 0.65714286 0.67142857 0.68571429 0.7 0.71428571 0.72857143 0.74285714 0.75714286 0.77142857 0.78571429 0.8 0.81428571 0.82857143 0.84285714 0.85714286 0.87142857 0.88571429 0.9 0.91428571 0.92857143 0.94285714 0.95714286 0.97142857 0.98571429 1 1 1 1 1 1
  arc A26 (-46.012, 2.6586) -> (-46.012, 3.3414) centre (-53.7044, 3) ccw
  spline S13 degree 5 poles (-46.012, 3.3414) (-46.0163, 3.3443) (-46.0249, 3.35) (-46.0379, 3.3586) (-46.0552, 3.37) (-46.0769, 3.3841) (-46.0986, 3.398) (-46.1203, 3.4117) (-46.1421, 3.4253) (-46.1639, 3.4388) (-46.1857, 3.452) (-46.2076, 3.4652) (-46.2295, 3.4781) (-46.2514, 3.4909) (-46.2734, 3.5036) (-46.2953, 3.516) (-46.3174, 3.5284) (-46.3394, 3.5405) (-46.3615, 3.5525) (-46.3836, 3.5643) (-46.4057, 3.576) (-46.4278, 3.5874) (-46.45, 3.5988) (-46.4722, 3.6099) (-46.4944, 3.6209) (-46.5167, 3.6317) (-46.5389, 3.6423) (-46.5612, 3.6527) (-46.5835, 3.663) (-46.6058, 3.6731) (-46.6281, 3.683) (-46.6505, 3.6928) (-46.6729, 3.7023) (-46.6952, 3.7117) (-46.7176, 3.7209) (-46.74, 3.7299) (-46.7625, 3.7387) (-46.7849, 3.7474) (-46.8073, 3.7558) (-46.8298, 3.764) (-46.8523, 3.7721) (-46.8747, 3.7799) (-46.8972, 3.7876) (-46.9197, 3.795) (-46.9422, 3.8023) (-46.9647, 3.8093) (-46.9872, 3.8162) (-47.0097, 3.8228) (-47.0322, 3.8292) (-47.0547, 3.8354) (-47.0772, 3.8414) (-47.0997, 3.8471) (-47.1221, 3.8526) (-47.1446, 3.8579) (-47.1671, 3.8629) (-47.1896, 3.8676) (-47.212, 3.8722) (-47.2345, 3.8765) (-47.2569, 3.8806) (-47.2794, 3.8845) (-47.3018, 3.888) (-47.3242, 3.8912) (-47.3465, 3.8939) (-47.3689, 3.8963) (-47.3912, 3.8984) (-47.4135, 3.9002) (-47.4358, 3.9019) (-47.458, 3.9033) (-47.4802, 3.9045) (-47.5023, 3.9052) (-47.5244, 3.9051) (-47.542, 3.9042) (-47.5551, 3.9029) (-47.5639, 3.9017) (-47.5682, 3.9011) knots -1 -1 -1 -1 -1 -1 -0.98571429 -0.97142857 -0.95714286 -0.94285714 -0.92857143 -0.91428571 -0.9 -0.88571429 -0.87142857 -0.85714286 -0.84285714 -0.82857143 -0.81428571 -0.8 -0.78571429 -0.77142857 -0.75714286 -0.74285714 -0.72857143 -0.71428571 -0.7 -0.68571429 -0.67142857 -0.65714286 -0.64285714 -0.62857143 -0.61428571 -0.6 -0.58571429 -0.57142857 -0.55714286 -0.54285714 -0.52857143 -0.51428571 -0.5 -0.48571429 -0.47142857 -0.45714286 -0.44285714 -0.42857143 -0.41428571 -0.4 -0.38571429 -0.37142857 -0.35714286 -0.34285714 -0.32857143 -0.31428571 -0.3 -0.28571429 -0.27142857 -0.25714286 -0.24285714 -0.22857143 -0.21428571 -0.2 -0.18571429 -0.17142857 -0.15714286 -0.14285714 -0.12857143 -0.11428571 -0.1 -0.08571429 -0.07142857 -0.05714286 -0.04285714 -0.02857143 -0.01428571 0 0 0 0 0 0
  line L13 (-47.5682, 3.9011) -> (-48.3356, 3.7884)
  arc A27 (-48.4488, 3.871) -> (-48.3356, 3.7884) centre (-48.3501, 3.8873) ccw
  arc A28 (-48.4488, 3.871) -> (-48.7174, 4.8735) centre (-53.7044, 3) ccw
  arc A29 (-48.6607, 5.0016) -> (-48.7174, 4.8735) centre (-48.6238, 4.9087) ccw
  line L14 (-48.6607, 5.0016) -> (-47.9398, 5.2877)
  spline S14 degree 5 poles (-47.9398, 5.2877) (-47.9357, 5.2894) (-47.9275, 5.2927) (-47.9155, 5.2982) (-47.8998, 5.3062) (-47.8807, 5.3171) (-47.8618, 5.3288) (-47.8432, 5.3409) (-47.8247, 5.3533) (-47.8062, 5.3658) (-47.7878, 5.3785) (-47.7695, 5.3915) (-47.7514, 5.4047) (-47.7334, 5.4183) (-47.7156, 5.4323) (-47.6979, 5.4465) (-47.6804, 5.4611) (-47.663, 5.4759) (-47.6458, 5.4908) (-47.6286, 5.506) (-47.6115, 5.5214) (-47.5945, 5.537) (-47.5777, 5.5527) (-47.561, 5.5687) (-47.5443, 5.585) (-47.5279, 5.6014) (-47.5115, 5.618) (-47.4952, 5.6348) (-47.479, 5.6518) (-47.463, 5.669) (-47.447, 5.6863) (-47.4311, 5.7038) (-47.4154, 5.7215) (-47.3997, 5.7394) (-47.3842, 5.7574) (-47.3688, 5.7756) (-47.3535, 5.794) (-47.3382, 5.8125) (-47.3231, 5.8312) (-47.3081, 5.8501) (-47.2932, 5.8691) (-47.2784, 5.8882) (-47.2637, 5.9075) (-47.2491, 5.927) (-47.2347, 5.9466) (-47.2203, 5.9664) (-47.206, 5.9863) (-47.1918, 6.0063) (-47.1778, 6.0265) (-47.1638, 6.0468) (-47.1499, 6.0673) (-47.1362, 6.0879) (-47.1225, 6.1087) (-47.109, 6.1295) (-47.0956, 6.1506) (-47.0822, 6.1717) (-47.069, 6.193) (-47.0559, 6.2144) (-47.0429, 6.2359) (-47.0299, 6.2576) (-47.0171, 6.2794) (-47.0044, 6.3013) (-46.9919, 6.3234) (-46.9794, 6.3456) (-46.967, 6.3679) (-46.9547, 6.3903) (-46.9426, 6.4128) (-46.9305, 6.4355) (-46.9186, 6.4583) (-46.9067, 6.4812) (-46.895, 6.5042) (-46.8857, 6.5227) (-46.8787, 6.5366) (-46.8742, 6.5459) (-46.8719, 6.5506) knots 0 0 0 0 0 0 0.01428571 0.02857143 0.04285714 0.05714286 0.07142857 0.08571429 0.1 0.11428571 0.12857143 0.14285714 0.15714286 0.17142857 0.18571429 0.2 0.21428571 0.22857143 0.24285714 0.25714286 0.27142857 0.28571429 0.3 0.31428571 0.32857143 0.34285714 0.35714286 0.37142857 0.38571429 0.4 0.41428571 0.42857143 0.44285714 0.45714286 0.47142857 0.48571429 0.5 0.51428571 0.52857143 0.54285714 0.55714286 0.57142857 0.58571429 0.6 0.61428571 0.62857143 0.64285714 0.65714286 0.67142857 0.68571429 0.7 0.71428571 0.72857143 0.74285714 0.75714286 0.77142857 0.78571429 0.8 0.81428571 0.82857143 0.84285714 0.85714286 0.87142857 0.88571429 0.9 0.91428571 0.92857143 0.94285714 0.95714286 0.97142857 0.98571429 1 1 1 1 1 1
  arc A30 (-46.8719, 6.5506) -> (-47.2132, 7.1419) centre (-53.7044, 3) ccw
  spline S15 degree 5 poles (-47.2132, 7.1419) (-47.2184, 7.1422) (-47.2288, 7.1429) (-47.2443, 7.1438) (-47.265, 7.145) (-47.2908, 7.1464) (-47.3165, 7.1476) (-47.3422, 7.1486) (-47.3679, 7.1495) (-47.3935, 7.1502) (-47.419, 7.1508) (-47.4445, 7.1513) (-47.47, 7.1515) (-47.4954, 7.1516) (-47.5207, 7.1516) (-47.546, 7.1514) (-47.5712, 7.1511) (-47.5964, 7.1506) (-47.6215, 7.1499) (-47.6465, 7.1491) (-47.6715, 7.1481) (-47.6964, 7.147) (-47.7213, 7.1457) (-47.7461, 7.1443) (-47.7708, 7.1427) (-47.7955, 7.1409) (-47.8201, 7.139) (-47.8446, 7.1369) (-47.869, 7.1346) (-47.8934, 7.1322) (-47.9177, 7.1297) (-47.9419, 7.1269) (-47.9661, 7.124) (-47.9901, 7.1209) (-48.0141, 7.1177) (-48.038, 7.1143) (-48.0619, 7.1107) (-48.0856, 7.107) (-48.1093, 7.1031) (-48.1328, 7.099) (-48.1563, 7.0947) (-48.1797, 7.0903) (-48.203, 7.0857) (-48.2262, 7.0809) (-48.2493, 7.0759) (-48.2723, 7.0708) (-48.2952, 7.0654) (-48.318, 7.0599) (-48.3407, 7.0542) (-48.3633, 7.0483) (-48.3857, 7.0423) (-48.4081, 7.036) (-48.4303, 7.0295) (-48.4524, 7.0228) (-48.4744, 7.0159) (-48.4962, 7.0088) (-48.5179, 7.0015) (-48.5396, 6.994) (-48.5611, 6.9864) (-48.5824, 6.9785) (-48.6036, 6.9703) (-48.6246, 6.9619) (-48.6453, 6.9531) (-48.6659, 6.944) (-48.6862, 6.9346) (-48.7064, 6.9251) (-48.7265, 6.9154) (-48.7465, 6.9055) (-48.7663, 6.8954) (-48.7859, 6.8849) (-48.8049, 6.8738) (-48.8197, 6.8642) (-48.8304, 6.8565) (-48.8374, 6.8512) (-48.8409, 6.8484) knots -1 -1 -1 -1 -1 -1 -0.98571429 -0.97142857 -0.95714286 -0.94285714 -0.92857143 -0.91428571 -0.9 -0.88571429 -0.87142857 -0.85714286 -0.84285714 -0.82857143 -0.81428571 -0.8 -0.78571429 -0.77142857 -0.75714286 -0.74285714 -0.72857143 -0.71428571 -0.7 -0.68571429 -0.67142857 -0.65714286 -0.64285714 -0.62857143 -0.61428571 -0.6 -0.58571429 -0.57142857 -0.55714286 -0.54285714 -0.52857143 -0.51428571 -0.5 -0.48571429 -0.47142857 -0.45714286 -0.44285714 -0.42857143 -0.41428571 -0.4 -0.38571429 -0.37142857 -0.35714286 -0.34285714 -0.32857143 -0.31428571 -0.3 -0.28571429 -0.27142857 -0.25714286 -0.24285714 -0.22857143 -0.21428571 -0.2 -0.18571429 -0.17142857 -0.15714286 -0.14285714 -0.12857143 -0.11428571 -0.1 -0.08571429 -0.07142857 -0.05714286 -0.04285714 -0.02857143 -0.01428571 0 0 0 0 0 0
  line L15 (-48.8409, 6.8484) -> (-49.4491, 6.3672)
  arc A31 (-49.5884, 6.3821) -> (-49.4491, 6.3672) centre (-49.5111, 6.4456) ccw
  arc A32 (-49.5884, 6.3821) -> (-50.3223, 7.116) centre (-53.7044, 3) ccw
  arc A33 (-50.3372, 7.2553) -> (-50.3223, 7.116) centre (-50.2588, 7.1933) ccw
  line L16 (-50.3372, 7.2553) -> (-49.856, 7.8635)
  spline S16 degree 5 poles (-49.856, 7.8635) (-49.8532, 7.867) (-49.8479, 7.874) (-49.8402, 7.8847) (-49.8306, 7.8995) (-49.8195, 7.9185) (-49.809, 7.9381) (-49.7989, 7.9579) (-49.789, 7.9779) (-49.7793, 7.998) (-49.7697, 8.0182) (-49.7604, 8.0385) (-49.7513, 8.0591) (-49.7425, 8.0798) (-49.7341, 8.1008) (-49.7259, 8.122) (-49.718, 8.1433) (-49.7104, 8.1648) (-49.7029, 8.1864) (-49.6956, 8.2082) (-49.6885, 8.23) (-49.6816, 8.252) (-49.6749, 8.2741) (-49.6684, 8.2963) (-49.6621, 8.3187) (-49.656, 8.3411) (-49.6502, 8.3637) (-49.6445, 8.3864) (-49.639, 8.4092) (-49.6336, 8.4321) (-49.6285, 8.4551) (-49.6235, 8.4782) (-49.6187, 8.5014) (-49.6141, 8.5247) (-49.6097, 8.5481) (-49.6054, 8.5716) (-49.6013, 8.5951) (-49.5974, 8.6188) (-49.5937, 8.6425) (-49.5901, 8.6664) (-49.5867, 8.6903) (-49.5834, 8.7143) (-49.5804, 8.7383) (-49.5775, 8.7625) (-49.5747, 8.7867) (-49.5722, 8.811) (-49.5697, 8.8354) (-49.5675, 8.8598) (-49.5654, 8.8843) (-49.5635, 8.9089) (-49.5617, 8.9336) (-49.5601, 8.9583) (-49.5587, 8.9831) (-49.5574, 9.008) (-49.5562, 9.0329) (-49.5553, 9.0579) (-49.5545, 9.0829) (-49.5538, 9.108) (-49.5533, 9.1332) (-49.553, 9.1584) (-49.5528, 9.1837) (-49.5527, 9.209) (-49.5529, 9.2344) (-49.5531, 9.2599) (-49.5536, 9.2854) (-49.5541, 9.3109) (-49.5549, 9.3365) (-49.5558, 9.3622) (-49.5568, 9.3879) (-49.558, 9.4136) (-49.5593, 9.4394) (-49.5605, 9.4601) (-49.5615, 9.4756) (-49.5622, 9.486) (-49.5625, 9.4911) knots 0 0 0 0 0 0 0.01428571 0.02857143 0.04285714 0.05714286 0.07142857 0.08571429 0.1 0.11428571 0.12857143 0.14285714 0.15714286 0.17142857 0.18571429 0.2 0.21428571 0.22857143 0.24285714 0.25714286 0.27142857 0.28571429 0.3 0.31428571 0.32857143 0.34285714 0.35714286 0.37142857 0.38571429 0.4 0.41428571 0.42857143 0.44285714 0.45714286 0.47142857 0.48571429 0.5 0.51428571 0.52857143 0.54285714 0.55714286 0.57142857 0.58571429 0.6 0.61428571 0.62857143 0.64285714 0.65714286 0.67142857 0.68571429 0.7 0.71428571 0.72857143 0.74285714 0.75714286 0.77142857 0.78571429 0.8 0.81428571 0.82857143 0.84285714 0.85714286 0.87142857 0.88571429 0.9 0.91428571 0.92857143 0.94285714 0.95714286 0.97142857 0.98571429 1 1 1 1 1 1
  arc A34 (-49.5625, 9.4911) -> (-50.1538, 9.8325) centre (-53.7044, 3) ccw
  spline S17 degree 5 poles (-50.1538, 9.8325) (-50.1585, 9.8302) (-50.1678, 9.8256) (-50.1817, 9.8187) (-50.2002, 9.8094) (-50.2232, 9.7977) (-50.2461, 9.7858) (-50.2689, 9.7739) (-50.2916, 9.7618) (-50.3141, 9.7497) (-50.3365, 9.7374) (-50.3588, 9.725) (-50.381, 9.7125) (-50.403, 9.6999) (-50.425, 9.6872) (-50.4468, 9.6744) (-50.4684, 9.6615) (-50.49, 9.6485) (-50.5114, 9.6354) (-50.5327, 9.6222) (-50.5538, 9.6088) (-50.5749, 9.5954) (-50.5957, 9.5819) (-50.6165, 9.5682) (-50.6371, 9.5545) (-50.6576, 9.5406) (-50.6779, 9.5266) (-50.6981, 9.5126) (-50.7181, 9.4984) (-50.738, 9.4841) (-50.7578, 9.4697) (-50.7774, 9.4552) (-50.7969, 9.4407) (-50.8162, 9.426) (-50.8353, 9.4112) (-50.8543, 9.3963) (-50.8732, 9.3813) (-50.8919, 9.3661) (-50.9104, 9.3509) (-50.9288, 9.3356) (-50.947, 9.3202) (-50.965, 9.3046) (-50.9829, 9.289) (-51.0006, 9.2732) (-51.0181, 9.2574) (-51.0354, 9.2414) (-51.0526, 9.2254) (-51.0696, 9.2092) (-51.0864, 9.1929) (-51.103, 9.1765) (-51.1194, 9.16) (-51.1356, 9.1434) (-51.1517, 9.1267) (-51.1674, 9.1098) (-51.183, 9.0929) (-51.1984, 9.0758) (-51.2135, 9.0586) (-51.2285, 9.0413) (-51.2433, 9.024) (-51.2579, 9.0065) (-51.2721, 8.9888) (-51.2861, 8.971) (-51.2997, 8.953) (-51.3129, 8.9349) (-51.3258, 8.9166) (-51.3386, 8.8982) (-51.3511, 8.8797) (-51.3635, 8.8612) (-51.3756, 8.8426) (-51.3873, 8.8237) (-51.3982, 8.8046) (-51.4062, 8.7889) (-51.4117, 8.7768) (-51.415, 8.7687) (-51.4167, 8.7646) knots -1 -1 -1 -1 -1 -1 -0.98571429 -0.97142857 -0.95714286 -0.94285714 -0.92857143 -0.91428571 -0.9 -0.88571429 -0.87142857 -0.85714286 -0.84285714 -0.82857143 -0.81428571 -0.8 -0.78571429 -0.77142857 -0.75714286 -0.74285714 -0.72857143 -0.71428571 -0.7 -0.68571429 -0.67142857 -0.65714286 -0.64285714 -0.62857143 -0.61428571 -0.6 -0.58571429 -0.57142857 -0.55714286 -0.54285714 -0.52857143 -0.51428571 -0.5 -0.48571429 -0.47142857 -0.45714286 -0.44285714 -0.42857143 -0.41428571 -0.4 -0.38571429 -0.37142857 -0.35714286 -0.34285714 -0.32857143 -0.31428571 -0.3 -0.28571429 -0.27142857 -0.25714286 -0.24285714 -0.22857143 -0.21428571 -0.2 -0.18571429 -0.17142857 -0.15714286 -0.14285714 -0.12857143 -0.11428571 -0.1 -0.08571429 -0.07142857 -0.05714286 -0.04285714 -0.02857143 -0.01428571 0 0 0 0 0 0
  line L17 (-51.4167, 8.7646) -> (-51.7028, 8.0437)
  arc A35 (-51.8309, 7.987) -> (-51.7028, 8.0437) centre (-51.7957, 8.0806) ccw
  arc A36 (-51.8309, 7.987) -> (-52.8334, 8.2556) centre (-53.7044, 3) ccw
  arc A37 (-52.916, 8.3688) -> (-52.8334, 8.2556) centre (-52.8171, 8.3543) ccw
  line L18 (-52.916, 8.3688) -> (-52.8033, 9.1362)
  spline S18 degree 5 poles (-52.8033, 9.1362) (-52.8027, 9.1405) (-52.8015, 9.1493) (-52.8002, 9.1624) (-52.7993, 9.18) (-52.7992, 9.202) (-52.7999, 9.2242) (-52.8011, 9.2464) (-52.8025, 9.2686) (-52.8042, 9.2909) (-52.806, 9.3132) (-52.808, 9.3355) (-52.8104, 9.3578) (-52.8132, 9.3802) (-52.8164, 9.4026) (-52.8199, 9.425) (-52.8238, 9.4474) (-52.8279, 9.4699) (-52.8322, 9.4923) (-52.8368, 9.5148) (-52.8415, 9.5373) (-52.8465, 9.5598) (-52.8518, 9.5822) (-52.8573, 9.6047) (-52.863, 9.6272) (-52.869, 9.6497) (-52.8752, 9.6722) (-52.8816, 9.6947) (-52.8882, 9.7172) (-52.8951, 9.7397) (-52.9021, 9.7622) (-52.9093, 9.7847) (-52.9168, 9.8072) (-52.9244, 9.8297) (-52.9323, 9.8521) (-52.9403, 9.8746) (-52.9486, 9.8971) (-52.957, 9.9195) (-52.9657, 9.9419) (-52.9745, 9.9644) (-52.9835, 9.9868) (-52.9927, 10.0092) (-53.0021, 10.0315) (-53.0116, 10.0539) (-53.0213, 10.0763) (-53.0313, 10.0986) (-53.0414, 10.1209) (-53.0516, 10.1432) (-53.0621, 10.1655) (-53.0727, 10.1877) (-53.0835, 10.21) (-53.0945, 10.2322) (-53.1056, 10.2544) (-53.117, 10.2765) (-53.1284, 10.2987) (-53.1401, 10.3208) (-53.1519, 10.3429) (-53.1639, 10.365) (-53.176, 10.387) (-53.1883, 10.409) (-53.2008, 10.431) (-53.2135, 10.453) (-53.2263, 10.4749) (-53.2392, 10.4968) (-53.2523, 10.5187) (-53.2656, 10.5405) (-53.2791, 10.5623) (-53.2927, 10.5841) (-53.3064, 10.6058) (-53.3203, 10.6275) (-53.3344, 10.6492) (-53.3458, 10.6665) (-53.3544, 10.6795) (-53.3601, 10.6881) (-53.363, 10.6924) knots 0 0 0 0 0 0 0.01428571 0.02857143 0.04285714 0.05714286 0.07142857 0.08571429 0.1 0.11428571 0.12857143 0.14285714 0.15714286 0.17142857 0.18571429 0.2 0.21428571 0.22857143 0.24285714 0.25714286 0.27142857 0.28571429 0.3 0.31428571 0.32857143 0.34285714 0.35714286 0.37142857 0.38571429 0.4 0.41428571 0.42857143 0.44285714 0.45714286 0.47142857 0.48571429 0.5 0.51428571 0.52857143 0.54285714 0.55714286 0.57142857 0.58571429 0.6 0.61428571 0.62857143 0.64285714 0.65714286 0.67142857 0.68571429 0.7 0.71428571 0.72857143 0.74285714 0.75714286 0.77142857 0.78571429 0.8 0.81428571 0.82857143 0.84285714 0.85714286 0.87142857 0.88571429 0.9 0.91428571 0.92857143 0.94285714 0.95714286 0.97142857 0.98571429 1 1 1 1 1 1
  arc A38 (-53.363, 10.6924) -> (-54.0458, 10.6924) centre (-53.7044, 3) ccw
  spline S19 degree 5 poles (-54.0458, 10.6924) (-54.0487, 10.6881) (-54.0544, 10.6795) (-54.063, 10.6665) (-54.0744, 10.6492) (-54.0885, 10.6275) (-54.1024, 10.6058) (-54.1161, 10.5841) (-54.1297, 10.5623) (-54.1432, 10.5405) (-54.1564, 10.5187) (-54.1696, 10.4968) (-54.1825, 10.4749) (-54.1953, 10.453) (-54.208, 10.431) (-54.2204, 10.409) (-54.2327, 10.387) (-54.2449, 10.365) (-54.2569, 10.3429) (-54.2687, 10.3208) (-54.2803, 10.2987) (-54.2918, 10.2765) (-54.3031, 10.2544) (-54.3143, 10.2322) (-54.3253, 10.21) (-54.3361, 10.1877) (-54.3467, 10.1655) (-54.3571, 10.1432) (-54.3674, 10.1209) (-54.3775, 10.0986) (-54.3874, 10.0763) (-54.3972, 10.0539) (-54.4067, 10.0315) (-54.4161, 10.0092) (-54.4253, 9.9868) (-54.4343, 9.9644) (-54.4431, 9.9419) (-54.4517, 9.9195) (-54.4602, 9.8971) (-54.4684, 9.8746) (-54.4765, 9.8521) (-54.4843, 9.8297) (-54.492, 9.8072) (-54.4994, 9.7847) (-54.5067, 9.7622) (-54.5137, 9.7397) (-54.5205, 9.7172) (-54.5272, 9.6947) (-54.5336, 9.6722) (-54.5398, 9.6497) (-54.5458, 9.6272) (-54.5515, 9.6047) (-54.557, 9.5822) (-54.5622, 9.5598) (-54.5672, 9.5373) (-54.572, 9.5148) (-54.5766, 9.4923) (-54.5809, 9.4699) (-54.585, 9.4474) (-54.5889, 9.425) (-54.5924, 9.4026) (-54.5956, 9.3802) (-54.5983, 9.3578) (-54.6007, 9.3355) (-54.6028, 9.3132) (-54.6046, 9.2909) (-54.6063, 9.2686) (-54.6077, 9.2464) (-54.6089, 9.2242) (-54.6096, 9.202) (-54.6095, 9.18) (-54.6085, 9.1624) (-54.6072, 9.1493) (-54.6061, 9.1405) (-54.6055, 9.1362) knots -1 -1 -1 -1 -1 -1 -0.98571429 -0.97142857 -0.95714286 -0.94285714 -0.92857143 -0.91428571 -0.9 -0.88571429 -0.87142857 -0.85714286 -0.84285714 -0.82857143 -0.81428571 -0.8 -0.78571429 -0.77142857 -0.75714286 -0.74285714 -0.72857143 -0.71428571 -0.7 -0.68571429 -0.67142857 -0.65714286 -0.64285714 -0.62857143 -0.61428571 -0.6 -0.58571429 -0.57142857 -0.55714286 -0.54285714 -0.52857143 -0.51428571 -0.5 -0.48571429 -0.47142857 -0.45714286 -0.44285714 -0.42857143 -0.41428571 -0.4 -0.38571429 -0.37142857 -0.35714286 -0.34285714 -0.32857143 -0.31428571 -0.3 -0.28571429 -0.27142857 -0.25714286 -0.24285714 -0.22857143 -0.21428571 -0.2 -0.18571429 -0.17142857 -0.15714286 -0.14285714 -0.12857143 -0.11428571 -0.1 -0.08571429 -0.07142857 -0.05714286 -0.04285714 -0.02857143 -0.01428571 0 0 0 0 0 0
  line L19 (-54.6055, 9.1362) -> (-54.4928, 8.3688)
  arc A39 (-54.5754, 8.2556) -> (-54.4928, 8.3688) centre (-54.5917, 8.3543) ccw
  arc A40 (-54.5754, 8.2556) -> (-55.5779, 7.987) centre (-53.7044, 3) ccw
  arc A41 (-55.706, 8.0437) -> (-55.5779, 7.987) centre (-55.6131, 8.0806) ccw
  line L20 (-55.706, 8.0437) -> (-55.9921, 8.7646)